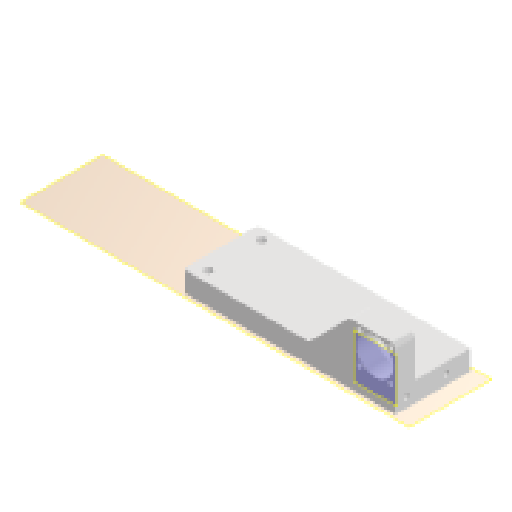
# Autodesk Inventor part: OT2-Gripper_base
Saved by Autodesk Inventor 2024.1 (Build 281209000, 209)
## iProperties
Created: 2024-09-05
Part Number: OT2-Gripper_base
Material: Generisch
Document SubType Name: Modeling
Designer: diederichbenedict
Density: 1 g/cm^3
Appearance: Vorgabe
Author: diederichbenedict
Autodesk Inventor part; units mm, degrees
ref_plane "YZ Plane" through (0, 0, 0) normal (1, 0, 0) x (0, 1, 0)
ref_plane "XZ Plane" through (0, 0, 0) normal (0, 1, 0) x (-1, 0, 0)
ref_plane "XY Plane" through (0, 0, 0) normal (0, 0, 1) x (1, 0, 0)
ref_plane "Arbeitsebene1" through (0, 0, 0) normal (0, 0, 1) x (1, 0, 0)
sketch "Skizze1" plane through (0, 0, 0) normal (0, 0, 1) x (1, 0, 0)
  line L0 (-106.15, 0) -> (-106.15, 8) projected
  line L1 (0, 0) -> (-106.15, 0) projected
  line L2 (0, 0) -> (0, 37.5) projected
  line L3 (0, 37.5) -> (-176.65, 37.5) projected
  line L4 (-176.65, 0) -> (-176.65, 37.5) projected
  line L5 (-137.15, 0) -> (-176.65, 0) projected
  line L6 (-137.15, 8) -> (-137.15, 0) projected
  arc A0 (-135.15, 10) -> (-137.15, 8) centre (-135.15, 8) ccw projected
  line L7 (-108.15, 10) -> (-135.15, 10) projected
  arc A1 (-106.15, 8) -> (-108.15, 10) centre (-108.15, 8) ccw projected
  circle A2 centre (-99, 32.01) radius 1.9 construction
  arc A3 (-9.5, 2.18) -> (-9.5, 9.18) centre (-9.5, 5.68) ccw projected
  line L8 (-10.5, 2.18) -> (-9.5, 2.18) projected
  arc A4 (-10.5, 9.18) -> (-10.5, 2.18) centre (-10.5, 5.68) ccw projected
  line L9 (-9.5, 9.18) -> (-10.5, 9.18) projected
  circle A5 centre (-99, 5.68) radius 1.525 construction
  circle A6 centre (-99, 32.01) radius 1.4
  circle A7 centre (-99, 5.68) radius 1.4
  line L10 (-20.2, 0) -> (-20.2, -25.9) projected
  line L11 (0, 0) -> (0, -25.9) projected
  line L12 (-106.15, 37.5) -> (0, 37.5)
  line L13 (0, 37.5) -> (0, 0)
  line L14 (0, 0) -> (-106.15, 0)
  line L15 (-106.15, 0) -> (-106.15, 37.5)
  dimension "d0" = 2.8
  dimension "d1" = 2.8
  constraints: 8 end point, 2 centre point, 2 coincident, 2 parallel, 1 horizontal, 1 perpendicular, 1 point on line
  measures "d0" diameter of A6
  measures "d1" diameter of A7
extrude "Extrusion1" add sketch "Skizze1" along normal blind 10 contours L0 L15 L3 L2 L1
ref_plane "Arbeitsebene2" through (0, 0, 25.2) normal (0, 1, 0) x (0, 0, -1)
sketch "Skizze2" plane through (0, 0, 25.2) normal (0, 1, 0) x (0, 0, -1)
  line L0 (-5, 17.9) -> (-5, 2.3) projected
  arc A0 (-5, 2.3) -> (-2.7, 0) centre (-2.7, 2.3) ccw projected
  line L1 (-2.7, 0) -> (12.9, 0) projected
  arc A1 (12.9, 0) -> (15.2, 2.3) centre (12.9, 2.3) ccw projected
  line L2 (15.2, 2.3) -> (15.2, 17.9) projected
  arc A2 (15.2, 17.9) -> (12.9, 20.2) centre (12.9, 17.9) ccw projected
  line L3 (12.9, 20.2) -> (-2.7, 20.2) projected
  arc A3 (-2.7, 20.2) -> (-5, 17.9) centre (-2.7, 17.9) ccw projected
  circle A4 centre (5.1, 10.1) radius 8 projected
  circle A5 centre (-2.6, 2.4) radius 1 projected
  circle A6 centre (12.8, 2.4) radius 1 projected
  circle A7 centre (12.8, 17.8) radius 1 projected
  circle A8 centre (-2.6, 17.8) radius 1 projected
  line L4 (-5, 17.9) -> (-5, 22.9389)
  line L5 (-5, 22.9389) -> (15.2, 43.1389)
  line L6 (15.2, 106.15) -> (15.2, 0) projected
  line L7 (15.2, 0) -> (15.2, 2.3)
  line L8 (15.2, 0) -> (-5, 0)
  line L9 (-5, 0) -> (-5, 20.2)
  line L10 (-5, 20.2) -> (15.2, 20.2)
  line L11 (15.2, 20.2) -> (15.2, 0)
  point P0 (25.2, 0)
  point P1 (15.2, 20.2)
  point P2 (15.2, 17.9)
  point P3 (12.9, 0)
  point P4 (15.2, 2.3)
  dimension "d13" = 135
  constraints: 14 end point, 3 point on line, 2 parallel, 1 horizontal, 1 perpendicular, 1 vertical
  measures "d13" angle of L4 L5
extrude "Extrusion2" add sketch "Skizze2" along normal blind 10 contours A3 L3 A2 L2 A1 L1 A0 L0 | L4 L10 A3 | L10 L4 L5 L6 L3 | L10 L6 A2 | A1 L6 L8
sketch "Skizze3" plane through (-106.15, 37.5, 0) normal (0, 1, 0) x (1, 0, 0)
  circle A0 centre (96.05, -20.1) radius 8 projected
  circle A1 centre (88.35, -27.8) radius 1 projected
  circle A2 centre (88.35, -12.4) radius 1 projected
  circle A3 centre (103.75, -27.8) radius 1 projected
  circle A4 centre (103.75, -12.4) radius 1 projected
  circle A5 centre (96.05, -20.1) radius 9
  circle A6 centre (88.35, -27.8) radius 1.25
  circle A7 centre (103.75, -27.8) radius 1.25
  circle A8 centre (103.75, -12.4) radius 1.25
  circle A9 centre (88.35, -12.4) radius 1.25
  point P0 (106.15, 0)
  point P1 (102.2136, -10)
  point P2 (89.8864, -10)
  dimension "d6" = 18
  dimension "d7" = 2.5
  dimension "d8" = 2.5
  dimension "d9" = 2.5
  dimension "d10" = 2.5
  constraints: 5 centre point, 5 coincident, 1 other
  measures "d6" diameter of A5
  measures "d7" diameter of A6
  measures "d8" diameter of A7
  measures "d9" diameter of A8
  measures "d10" diameter of A9
extrude "Extrusion3" cut sketch "Skizze3" against normal through all contours A0 | A1 | A2 | A3 | A4 | A5 | A6 | A7 | A8 | A9
fillet "Rundung1" radius 2 4 edges at (-22.9389, 5, 30.2) (-43.1389, 5, 10) (-106.15, 37.5, 5) (-106.15, 0, 5)
sketch "Skizze4" plane through (0, 0, 0) normal (1, 0, 0) x (0, 0, -1)
  circle A0 centre (-5, 25.5) radius 1.75 projected
  circle A1 centre (-5, 5.5) radius 1.75 projected
  point P0 (0, 0)
hole "Bohrung1" at (0, 25.5, 5) at (0, 5.5, 5) direction (-1, 0, 0) diameter 2.8 depth 15 tip angle 118
sketch "Skizze5" plane through (0, 0, 10) normal (0, 0, 1) x (1, 0, 0)
  arc A0 (-106.15, 2) -> (-104.15, 0) centre (-104.15, 2) ccw projected
  line L0 (-104.15, 0) -> (-43.9674, 0) projected
  line L1 (-43.9674, 10) -> (-43.9674, 0) projected
  line L2 (-43.9674, 10) -> (0, 10) projected
  line L3 (0, 10) -> (0, 37.5) projected
  line L4 (0, 37.5) -> (-104.15, 37.5) projected
  arc A1 (-104.15, 37.5) -> (-106.15, 35.5) centre (-104.15, 35.5) ccw projected
  line L5 (-106.15, 35.5) -> (-106.15, 2) projected
  circle A2 centre (-99, 32.01) radius 1.4 projected
  circle A3 centre (-99, 5.68) radius 1.4 projected
  point P0 (0, 0)
hole "Bohrung2" at (-99, 5.68, 10) at (-99, 32.01, 10) direction (0, 0, -1) diameter 4 depth 15 tip angle 118
